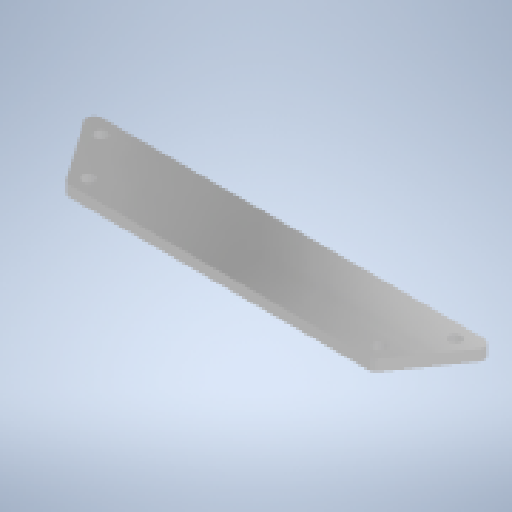
# Autodesk Inventor part: shield_side_side
Saved by Autodesk Inventor 2024.1 (Build 281209000, 209)
## iProperties
Created: 2024-02-14
Part Number: shield_side_side
Material: アルミニウム 6061
Document SubType Name: Modeling
Designer: hibik
Density: 2.7 g/cm^3
Appearance: アルミニウム - フラット
Author: hibik
Autodesk Inventor part; units mm, degrees
ref_plane "YZ Plane" through (0, 0, 0) normal (1, 0, 0) x (0, 1, 0)
ref_plane "XZ Plane" through (0, 0, 0) normal (0, 1, 0) x (-1, 0, 0)
ref_plane "XY Plane" through (0, 0, 0) normal (0, 0, 1) x (1, 0, 0)
sketch "スケッチ1" plane through (0, 0, 0) normal (0, 1, 0) x (-1, 0, 0)
  line L0 (55, 0) -> (0, 0)
  line L1 (0, 0) -> (0, -20)
  line L2 (0, -20) -> (55, -20)
  line L3 (55, -20) -> (55, 0)
  dimension "d0" = 20
  dimension "d1" = 55
  constraints: 8 end point, 2 parallel, 1 coincident, 1 horizontal, 1 perpendicular
  measures "d0" distance of L0.end L1.end
  measures "d1" distance of L0.start L0.end
extrude "押し出し1" add sketch "スケッチ1" along normal blind 1.5
sketch "スケッチ2" plane through (0, 0, 0) normal (0, -1, 0) x (1, 0, 0)
  line L0 (-7, -10.1005) -> (0, -20) projected
  line L1 (-7, -10.1005) -> (-48, -10.1005) projected
  line L2 (0, -20) -> (-55, -20) projected
  line L3 (-48, -10.1005) -> (-55, -20) projected
  line L4 (0, 0) -> (0, -20) projected
  line L5 (-55, 0) -> (0, 0) projected
  line L6 (-55, -20) -> (-55, 0) projected
  line L7 (0, -20) -> (-55, -20) projected
  point P0 (0, -20)
extrude "押し出し2" cut sketch "スケッチ2" against normal through all contours L1 L3 L6 L5 L4 L0
fillet "フィレット1" radius 1 4 edges at (-7, 0.75, -10.1005) (0, 0.75, -20) (-48, 0.75, -10.1005) (-55, 0.75, -20)
sketch "スケッチ3" plane through (0, 0, 0) normal (0, -1, 0) x (1, 0, 0)
  arc A0 (-53.8846, -18.4226) -> (-53.0681, -20) centre (-53.0681, -19) ccw projected
  line L0 (-1.9319, -20) -> (-53.0681, -20) projected
  arc A1 (-1.9319, -20) -> (-1.1154, -18.4226) centre (-1.9319, -19) ccw projected
  line L1 (-1.1154, -18.4226) -> (-6.7011, -10.5232) projected
  arc A2 (-6.7011, -10.5232) -> (-7.5176, -10.1005) centre (-7.5176, -11.1005) ccw projected
  line L2 (-7.5176, -10.1005) -> (-47.4824, -10.1005) projected
  arc A3 (-47.4824, -10.1005) -> (-48.2989, -10.5232) centre (-47.4824, -11.1005) ccw projected
  line L3 (-48.2989, -10.5232) -> (-53.8846, -18.4226) projected
  circle A4 centre (-46.9647, -12.1005) radius 0.8
  circle A5 centre (-8.0353, -12.1005) radius 0.8
  circle A6 centre (-3.8637, -18) radius 0.8
  circle A7 centre (-51.1363, -18) radius 0.8
  circle A8 centre (-27.5, 18.8909) radius 46.7105
  line L4 (-27.5, 18.8909) -> (-54.4683, -19.2481)
  line L5 (-27.5, 18.8909) -> (-0.5317, -19.2481)
  arc A9 (-53.8846, -18.4226) -> (-53.0681, -20) centre (-53.0681, -19) ccw projected
  line L6 (-27.5, 18.8909) -> (-49.0163, -22.569)
  line L7 (-27.5, 18.8909) -> (-43.1624, -25.1155)
  line L8 (-27.5, 18.8909) -> (-37.016, -26.84)
  line L9 (-27.5, 18.8909) -> (-30.6919, -27.7104)
  line L10 (-27.5, 18.8909) -> (-24.3081, -27.7104)
  line L11 (-27.5, 18.8909) -> (-17.984, -26.84)
  line L12 (-27.5, 18.8909) -> (-11.8376, -25.1155)
  line L13 (-27.5, 18.8909) -> (-5.9837, -22.569)
  line L14 (-46.9647, -12.1005) -> (-8.0353, -12.1005)
  line L15 (-51.1363, -18) -> (-3.8637, -18)
  line L16 (-46.9647, -12.1005) -> (-51.1363, -18)
  line L17 (-8.0353, -12.1005) -> (-3.8637, -18)
  circle A10 centre (-46.9647, -12.1005) radius 3.0011
  circle A11 centre (-51.1363, -18) radius 3.9863
  circle A12 centre (-8.0353, -12.1005) radius 3.0011
  circle A13 centre (-3.8637, -18) radius 3.9863
  line L18 (-43.5835, -12.1005) -> (-38.5302, -12.1005)
  point P0 (0, 0)
  point P1 (-14.37, -18)
  point P2 (-8.3548, -18)
  point P3 (-11.4165, -12.1005)
  point P4 (-16.4698, -12.1005)
  point P5 (-24.9732, -18)
  point P6 (-19.8235, -18)
  point P7 (-21.0511, -12.1005)
  point P8 (-25.3773, -12.1005)
  point P9 (-35.1765, -18)
  point P10 (-30.0268, -18)
  point P11 (-29.6227, -12.1005)
  point P12 (-33.9489, -12.1005)
  point P13 (-46.6452, -18)
  point P14 (-40.63, -18)
  dimension "d7" = 1.6
  dimension "d8" = 1.6
  dimension "d9" = 1.6
  dimension "d10" = 1.6
  dimension "d11" = 2
  dimension "d12" = 2
  dimension "d13" = 2
  dimension "d14" = 2
  dimension "d15" = 2
  dimension "d16" = 2
  dimension "d19" = 7.837
  dimension "d20" = 7.837
  dimension "d21" = 7.837
  dimension "d22" = 7.837
  dimension "d25" = 7.837
  dimension "d26" = 7.837
  dimension "d27" = 7.837
  dimension "d28" = 7.837
  dimension "d29" = 7.837
  constraints: 30 end point, 8 centre point, 4 coincident, 4 point on line, 4 tangent, 2 collinear, 2 horizontal, 2 horizontal alignment, 13 other
  measures "d7" diameter of A4
  measures "d8" diameter of A5
  measures "d9" diameter of A6
  measures "d10" diameter of A7
  measures "d11" distance from line of L2 L14.start
  measures "d12" distance from line of L3 L14.start
  measures "d13" distance from line of L1 L14.end
  measures "d14" distance from line of L0 L15.start
  measures "d15" distance from line of L3 L15.start
  measures "d16" distance from line of L1 L15.end
  measures "d19" angle of L4 L6
  measures "d20" angle of L6 L7
  measures "d21" angle of L7 L8
  measures "d22" angle of L8 L9
  measures "d25" angle of L11 L10
  measures "d26" angle of L12 L11
  measures "d27" angle of L13 L12
  measures "d28" angle of L10 L9
  measures "d29" angle of L5 L13
extrude "押し出し3" cut sketch "スケッチ3" against normal through all contours L16 L15 A7 | A7 L15 L16 | L16 L14 A4 | A4 L14 L16 | L6 L14 L7 L15 | L8 L14 L9 L15 | L14 L11 L15 L10 | L14 L13 L15 L12 | L14 L17 A5 | A5 L17 L14 | L17 L15 A6 | A6 L15 L17
fillet "フィレット2" radius 2 16 edges at (-43.5835, 0.75, -12.1005) (-38.5302, 0.75, -12.1005) (-46.6452, 0.75, -18) (-40.63, 0.75, -18) (-33.9489, 0.75, -12.1005) (-29.6227, 0.75, -12.1005) (-35.1765, 0.75, -18) (-30.0268, 0.75, -18) (-24.9732, 0.75, -18) (-25.3773, 0.75, -12.1005) (-21.0511, 0.75, -12.1005) (-19.8235, 0.75, -18) (-11.4165, 0.75, -12.1005) (-8.3548, 0.75, -18) (-14.37, 0.75, -18) (-16.4698, 0.75, -12.1005)
equation "\"d12\" = d11"
equation "\"d13\" = d11"
equation "\"d14\" = d11"
equation "\"d15\" = d11"
equation "\"d16\" = d11"
equation "\"d19\" = d29"
equation "\"d20\" = d19"
equation "\"d21\" = d19"
equation "\"d22\" = d19"
equation "\"d25\" = d19"
equation "\"d26\" = d19"
equation "\"d27\" = d19"
equation "\"d28\" = d19"
